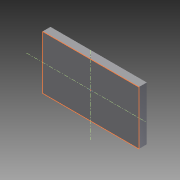
# Autodesk Inventor part: tv_42i
Saved by Autodesk Inventor 2011 (Build 150239000, 239)
## iProperties
Created: 2012-06-14
Part Number: tv_42i
Document SubType Name: Modeling
Designer: labuser
Density: 1 g/cm^3
Author: labuser
Autodesk Inventor part; units mm, degrees
ref_plane "YZ Plane" through (0, 0, 0) normal (1, 0, 0) x (0, 1, 0)
ref_plane "XZ Plane" through (0, 0, 0) normal (0, 1, 0) x (-1, 0, 0)
ref_plane "XY Plane" through (0, 0, 0) normal (0, 0, 1) x (1, 0, 0)
sketch "Sketch1" plane through (0, 0, 0) normal (0, 0, 1) x (1, 0, 0)
  line L0 (-466.09, -259.08) -> (466.09, -259.08)
  line L1 (466.09, -259.08) -> (466.09, 259.08)
  line L2 (466.09, 259.08) -> (-466.09, 259.08)
  line L3 (-466.09, 259.08) -> (-466.09, -259.08)
  point P0 (0, 0)
  dimension "d0" = 932.18
  dimension "d1" = 518.16
  constraints: 8 end point, 2 parallel, 1 horizontal, 1 perpendicular
  measures "d0" distance of L2.end L1.end
  measures "d1" distance of L1.end L0.end
extrude "Extrusion1" add sketch "Sketch1" along normal blind 76.2
sketch "Sketch3" plane through (0, 0, 76.2) normal (0, 0, 1) x (1, 0, 0)
  line L0 (466.09, -259.08) -> (-466.09, -259.08) projected
  line L1 (466.09, 259.08) -> (466.09, -259.08) projected
  line L2 (-466.09, 259.08) -> (466.09, 259.08) projected
  line L3 (-466.09, -259.08) -> (-466.09, 259.08) projected
  line L4 (-621.9572, 0) -> (531.0043, 0) construction
  line L5 (0, 337.0607) -> (0, -418.6507) construction
  point P0 (0, 0)
  point P1 (0, 0)
  constraints: 4 end point, 2 perpendicular, 1 coincident
body "Solid1"
